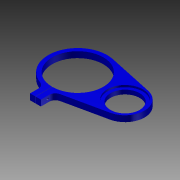
# Autodesk Inventor part: DispenserHolderArm
Saved by Autodesk Inventor 2012 SP1 (Build 160190100, 190)
## iProperties
Created: 2010-02-10
Part Number: DispenserHolderArm
Document SubType Name: Modeling
Designer: rconnaug
Density: 2.71 g/cm^3
Material: Aluminum-6061
Mass: 31.2115 g
Surface Area: 77.3456 cm^2
Volume: 11.5172 cm^3
Author: rconnaug
Autodesk Inventor part; units mm, degrees
ref_plane "YZ Plane" through (0, 0, 0) normal (1, 0, 0) x (0, 1, 0)
ref_plane "XZ Plane" through (0, 0, 0) normal (0, 1, 0) x (-1, 0, 0)
ref_plane "XY Plane" through (0, 0, 0) normal (0, 0, 1) x (1, 0, 0)
sketch "Sketch2" plane through (0, 0, 0) normal (0, 1, 0) x (-1, 0, 0)
  circle A0 centre (0, 0) radius 26.035
  line L0 (0, -51.0055) -> (0, 58.7294) construction
  line L1 (55.9949, 0) -> (-88.6658, 0) construction
  circle A1 centre (-48.175, 0) radius 17.9705
  arc A2 (-52.3622, 19.3778) -> (-52.3622, -19.3778) centre (-48.175, 0) ccw
  line L2 (-68, -23.8176) -> (-68, 24.095) construction
  line L3 (30, -24.7797) -> (30, 33.5235) construction
  line L4 (-6.3363, -29.3232) -> (-52.3622, -19.3778)
  line L5 (-6.3363, 29.3232) -> (-52.3622, 19.3778)
  line L6 (-5.5, 29.4915) -> (-5.5, 43.053)
  line L7 (-5.5, 43.053) -> (5.5, 43.053)
  line L8 (5.5, 43.053) -> (5.5, 29.4915)
  arc A3 (-6.3363, -29.3232) -> (5.5, 29.4915) centre (0, 0) ccw
  arc A4 (-5.5, 29.4915) -> (-6.3363, 29.3232) centre (0, 0) ccw
  point P0 (0, 43.053)
  point P1 (-66.1455, 0)
  point P2 (26.035, 0)
  dimension "d1" = 52.07
  dimension "d3" = 35.941
  dimension "d4" = 39.65
  dimension "d8" = 43.053
  dimension "d9" = 11
  dimension "d10" = 30
  dimension "d11" = 30
  dimension "d36" = 48.175
  constraints: 14 end point, 6 point on circle, 6 tangent, 4 point on line, 3 centre point, 3 coincident, 2 horizontal alignment, 2 parallel, 2 vertical, 1 horizontal, 1 midpoint, 1 perpendicular, 4 other
  measures "d4" diameter of A2
  measures "d8" distance from line of L7 point (0, 0)
  measures "d9" distance of L6.end L7.end
  measures "d10" radius of A3
  measures "d11" radius of A4
  measures "d36" distance of A2.centre point (0, 0)
extrude "Extrusion1" add sketch "Sketch2" along normal blind 6.1
sketch "Sketch3" plane through (5.5, 0, 43.053) normal (1, 0, 0) x (0, 0, -1)
  line L0 (13.5615, 6.1) -> (0, 6.1) projected
  line L1 (0, 0) -> (0, 6.1) projected
  point P0 (43.053, 0)
  point P1 (6.985, 3.05)
  dimension "d12" = 6.985
  dimension "d13" = 6.1
  dimension "d14" = 3.05
  measures "d12" distance from line of L1 point (6.985, 3.05)
  measures "d13" distance of L1.start L0.end
  measures "d14" distance from line of L0 point (6.985, 3.05)
hole "Hole1" at (5.5, 3.05, 36.068) direction (-1, 0, 0) diameter 2.159 depth 5.2578
sketch "Sketch4" plane through (0, 0, 0) normal (0, -1, 0) x (1, 0, 0)
  circle A0 centre (48.175, 0) radius 17.9705 projected
  arc A1 (52.3622, -19.3778) -> (52.3622, 19.3778) centre (48.175, 0) ccw projected
  circle A2 centre (48.175, 0) radius 14.85
  dimension "d22" = 29.7
  constraints: 1 centre point, 1 coincident
  measures "d22" diameter of A2
extrude "Extrusion2" add sketch "Sketch4" against normal blind 4.19
sketch "Sketch5" plane through (0, 6.1, 0) normal (0, 1, 0) x (1, 0, 0)
  circle A0 centre (0, 0) radius 26.035 projected
  line L0 (5.5, -43.053) -> (-5.5, -43.053) projected
  line L1 (-0.25, -43.053) -> (0.25, -43.053)
  line L2 (0.25, -43.053) -> (0.25, -26.0338)
  line L3 (0.25, -26.0338) -> (-0.25, -26.0338)
  line L4 (-0.25, -26.0338) -> (-0.25, -43.053)
  dimension "d25" = 0.5
  constraints: 8 end point, 2 parallel, 2 point on circle, 1 horizontal, 1 perpendicular, 1 point on line
  measures "d25" distance of L2.end L3.end
extrude "Extrusion3" cut sketch "Sketch5" against normal through all contours A0 L2 L0 L4
sketch "Sketch6" plane through (-5.5, 0, 29.4915) normal (-1, 0, 0) x (0, 0, 1)
  point P0 (-29.4915, 0)
  point P1 (6.5765, 3.05)
hole "Hole2" at (-5.5, 3.05, 36.068) direction (1, 0, 0) diameter 2.9464 end up to face face through (-0.25, 4.0667, 31.7069) facing (1, 0, 0) clearance for "Socket Head Cap Screw" size "#4" standard "Ansi Unified Screw Threads"
fillet "Fillet1" radius 6.35 2 edges at (-5.5, 3.05, 29.4915) (5.5, 3.05, 29.4915)
equation "\"d11\" = d10"
equation "\"d14\" = 0.5 * d13"
body "Solid1"
